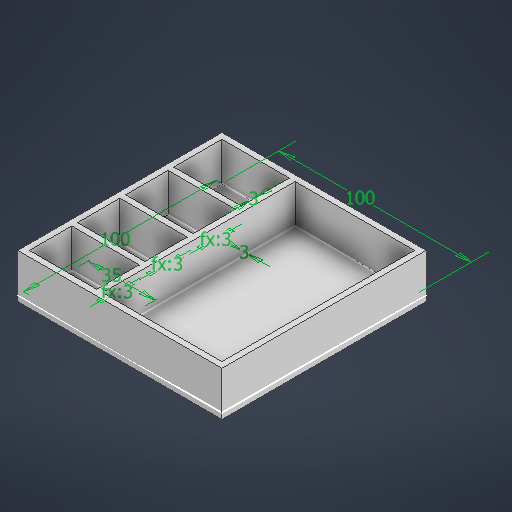
# Autodesk Inventor part: Cajita Organizadora
Saved by Autodesk Inventor 2026.1 (Build 301233000, 233)
## iProperties
Created: 2025-08-04
Part Number: Cajita Organizadora
Material: Genérico
Document SubType Name: Modeling
Designer: Laboratorio_sensores
Density: 1 g/cm^3
Appearance: Valor por defecto
Author: Laboratorio_sensores
Autodesk Inventor part; units mm, degrees
ref_plane "YZ Plane" through (0, 0, 0) normal (1, 0, 0) x (0, 1, 0)
ref_plane "XZ Plane" through (0, 0, 0) normal (0, 1, 0) x (-1, 0, 0)
ref_plane "XY Plane" through (0, 0, 0) normal (0, 0, 1) x (1, 0, 0)
sketch "Boceto1" plane through (0, 0, 0) normal (0, 1, 0) x (-1, 0, 0)
  line L0 (0, 0) -> (100, 0)
  line L1 (100, 0) -> (100, -100)
  line L2 (100, -100) -> (0, -100)
  line L3 (0, -100) -> (0, 0)
  line L4 (100, 0) -> (65, 0)
  line L5 (65, 0) -> (65, -50)
  line L6 (65, -100) -> (100, -100)
  line L7 (100, -100) -> (100, 0)
  line L8 (65, -50) -> (100, -50)
  line L9 (65, -50) -> (65, -100)
  line L10 (65, -25) -> (100, -25)
  line L11 (65, -75) -> (100, -75)
  line L12 (103, -103) -> (103, 3)
  line L13 (103, 3) -> (-3, 3)
  line L14 (-3, 3) -> (-3, -103)
  line L15 (-3, -103) -> (103, -103)
  line L16 (65, -72) -> (100, -72)
  line L17 (65, -47) -> (100, -47)
  line L18 (65, -22) -> (100, -22)
  line L19 (62, 0) -> (62, -100)
  dimension "d0" = 100
  dimension "d1" = 100
  dimension "d2" = 3
  dimension "d3" = 3
  dimension "d4" = 3
  dimension "d5" = 3
  dimension "d6" = 3
  dimension "d7" = 35
  constraints: 40 end point, 10 parallel, 9 point on line, 7 perpendicular, 3 horizontal, 3 midpoint, 3 other
  measures "d0" distance of L0.end L1.end
  measures "d1" distance of L1.end L2.end
  measures "d2" distance between parallel lines of L15 L2
  measures "d3" distance between parallel lines of L16 L11
  measures "d4" distance between parallel lines of L17 L8
  measures "d5" distance between parallel lines of L18 L10
  measures "d6" distance between parallel lines of L9 L19
  measures "d7" distance of L10.start L10.end
extrude "Extrusión1" add sketch "Boceto1" along normal blind 20 contours L0 L5 L9 L2 L19 | L18 L1 L10 L5 | L9 L16 L1 L11 | L17 L1 L8 L5 | L15 L14 L13 L12
extrude "Extrusión2" add sketch "Boceto1" against normal blind 3 contours L0 L19 L2 L3 | L0 L5 L9 L2 L19 | L0 L1 L18 L5 | L18 L1 L10 L5 | L9 L11 L1 L2 | L10 L1 L17 L5 | L9 L16 L1 L11 | L17 L1 L8 L5 | L9 L8 L1 L16 | L15 L14 L13 L12
equation "\"d3\" = d2"
equation "\"d4\" = d3"
equation "\"d5\" = d2"
